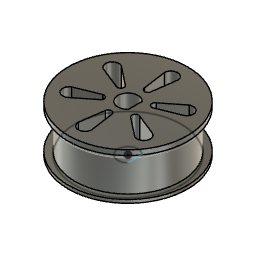
Maus_Komplettaufbau v3 (Autodesk Fusion 360 archive; units mm, degrees)
design "Wheel_v1"
Autodesk Fusion 360 part; units mm, degrees
sketch "Skizze1" plane through (0, 0, 0) normal (0, 0, 1) x (1, 0, 0)
  line L0 (1.05, 0) -> (1.05, 1.0712)
  line L1 (1.05, 0) -> (1.05, -1.0712)
  arc A0 (1.05, 1.0712) -> (1.05, -1.0712) centre (0, 0) ccw
  circle A1 centre (0, 0) radius 8
  dimension "d1" = 3
  dimension "d2" = 1.05
  dimension "d5" = 16
  constraint coincident A0.centre A1.centre
  measures "d1" diameter of A0
  measures "d2" distance of A0.centre L0.start
  measures "d5" diameter of A1
sketch "Skizze2" plane through (0, 0, 0) normal (0, 0, 1) x (1, 0, 0)
extrude "Extrusion2" add sketch "Skizze1" along normal blind 6
sketch "Skizze3" plane through (0, 0, 6) normal (0, 0, 1) x (-1, 0, 0)
  line L0 (-1.05, -1.0712) -> (-1.05, 1.0712)
  arc A0 (-1.05, -1.0712) -> (-1.05, 1.0712) centre (0, 0) ccw
  circle A1 centre (0, 0) radius 8
  line L1 (0.5, -3) -> (1, -6.5)
  line L2 (-1, -6.4999) -> (-0.4951, -2.93)
  arc A2 (-0.9608, -6.2227) -> (0.96, -6.22) centre (0, -6.5) ccw
  arc A3 (0.5, -3) -> (-0.4951, -2.93) centre (0, -3) ccw
  constraint coincident L1.end A2
  constraint coincident L2.start A2
  constraint tangent L2 A3
  constraint coincident L1 A2.end
  constraint coincident L2 A2.start
extrude "Extrusion3" cut sketch "Skizze3" against normal blind 6 contours L1 L2 A2 A3
pattern_circular "C-Anordnung1" count 6 over 360 about axis through (0, 0, 1.75) along (0, 0, 1) of "Extrusion3"
sketch "Skizze4" plane through (0, 0, 0) normal (0, 1, 0) x (1, 0, 0)
  line L0 (8, 0) -> (9, 0)
  line L1 (9, 0) -> (9, -0.5)
  line L2 (9, -0.5) -> (8, -0.5)
  line L3 (8, -0.5) -> (8, 0)
  line L4 (8, -6) -> (9, -6)
  line L5 (9, -6) -> (9, -5.5)
  line L6 (9, -5.5) -> (8, -5.5)
  line L7 (8, -5.5) -> (8, -6)
  constraint horizontal L0
  constraint vertical L1
  constraint horizontal L2
  constraint vertical L3
  constraint horizontal L4
  constraint vertical L5
  constraint horizontal L6
  constraint vertical L7
revolve "Drehen1" add sketch "Skizze4" angle 360 about axis through (0, 0, 1.75) along (0, 0, 1)
sketch "Skizze5" plane through (0, 0, 6) normal (0, 0, 1) x (-1, 0, 0)
  circle A0 centre (0, 0) radius 9
  arc A1 (-2.3481, -1.933) -> (-2.785, -1.0362) centre (-2.5981, -1.5) ccw
  line L0 (-2.3481, -1.933) -> (-5.1292, -4.116)
  arc A2 (-6.1291, -2.3839) -> (-5.1292, -4.116) centre (-5.6292, -3.25) ccw
  line L1 (-6.1291, -2.3839) -> (-2.785, -1.0362)
  arc A3 (-2.8481, 1.067) -> (-2.2899, 1.8937) centre (-2.5981, 1.5) ccw
  line L2 (-2.8481, 1.067) -> (-6.1292, 2.384)
  arc A4 (-5.1291, 4.116) -> (-6.1292, 2.384) centre (-5.6292, 3.25) ccw
  line L3 (-5.1291, 4.116) -> (-2.2899, 1.8937)
  arc A5 (-0.5, 3) -> (0.4951, 2.93) centre (0, 3) ccw
  line L4 (-0.5, 3) -> (-1, 6.5)
  arc A6 (1, 6.4999) -> (-1, 6.5) centre (0, 6.5) ccw
  line L5 (1, 6.4999) -> (0.4951, 2.93)
  arc A7 (2.3481, 1.933) -> (2.785, 1.0362) centre (2.5981, 1.5) ccw
  line L6 (2.3481, 1.933) -> (5.1292, 4.116)
  arc A8 (6.1291, 2.3839) -> (5.1292, 4.116) centre (5.6292, 3.25) ccw
  line L7 (6.1291, 2.3839) -> (2.785, 1.0362)
  arc A9 (2.8481, -1.067) -> (2.2899, -1.8937) centre (2.5981, -1.5) ccw
  line L8 (2.8481, -1.067) -> (6.1292, -2.384)
  arc A10 (5.1291, -4.116) -> (6.1292, -2.384) centre (5.6292, -3.25) ccw
  line L9 (5.1291, -4.116) -> (2.2899, -1.8937)
  arc A11 (0.5, -3) -> (-0.4951, -2.93) centre (0, -3) ccw
  line L10 (0.5, -3) -> (1, -6.5)
  arc A12 (-1, -6.4999) -> (1, -6.5) centre (0, -6.5) ccw
  line L11 (-1, -6.4999) -> (-0.4951, -2.93)
  line L12 (-1.05, -1.0712) -> (-1.05, 1.0712)
  arc A13 (-1.05, -1.0712) -> (-1.05, 1.0712) centre (0, 0) ccw
  line L13 (-1.1, 0) -> (-1.1, -1.0562)
  line L14 (-1.1, 0) -> (-1.1, 1.0562)
  arc A14 (-1.1, -1.0562) -> (-1.1, 1.0562) centre (0, 0) ccw
  dimension "d13" = 3.05
  constraint concentric A0 A14
  measures "d13" diameter of A14
extrude "Extrusion4" cut sketch "Skizze5" against normal blind 6 contours L13 L14 A14
extrude "Extrusion5" add 2 faces at (8.6332, -0.4471, 6) (5.0354, -0.3557, 6) along direction (0, 0, 1) blind 1
fillet "Abrundung1" radius 0.75 1 edges at (-8.3909, -3.2545, 5.5)

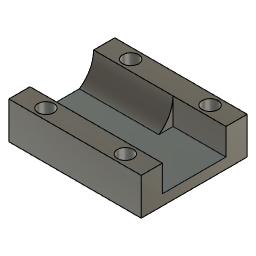
design "Motorhalter_v1"
Autodesk Fusion 360 part; units mm, degrees
sketch "Skizze1" plane through (0, 0, 0) normal (0, 0, 1) x (1, 0, 0)
  line L0 (0, 0) -> (-25, 0)
  line L1 (-25, 0) -> (-25, 20)
  line L2 (-25, 20) -> (0, 20)
  line L3 (0, 20) -> (0, 0)
  constraint horizontal L0
  constraint vertical L1
  constraint horizontal L2
  constraint vertical L3
  constraint coincident L0.start L3.end
extrude "Extrusion1" add sketch "Skizze1" along normal blind 7
sketch "Skizze2" plane through (0, 0, 0) normal (1, 0, 0) x (0, 1, 0)
  line L0 (0, 0) -> (20, 0)
  line L1 (20, 0) -> (20, 7)
  line L2 (20, 7) -> (0, 7)
  line L3 (0, 7) -> (0, 0)
  line L4 (10, 7) -> (4, 7)
  line L5 (4, 7) -> (4, 2)
  line L6 (4, 2) -> (16, 2)
  line L7 (16, 2) -> (16, 7)
  line L8 (16, 7) -> (10, 7)
  constraint midpoint L2 L4.start
  constraint coincident L2 L4.end
  constraint perpendicular L4 L5
  constraint coincident L2 L7.end
  constraint perpendicular L2 L7
extrude "Extrusion2" cut sketch "Skizze2" against normal blind 10 contours L2 L4 L5 L6 L7 L8
sketch "Skizze3" plane through (-10, 0, 0) normal (1, 0, 0) x (0, 1, 0)
  line L0 (16, 7) -> (4, 7)
  line L1 (4, 7) -> (4, 2)
  line L2 (4, 2) -> (16, 2)
  line L3 (16, 2) -> (16, 7)
  line L4 (6.6834, 2) -> (13.3166, 2)
  line L5 (16, 7) -> (4, 7)
  arc A0 (4, 7) -> (6.6834, 2) centre (10, 7) ccw
  arc A1 (13.3166, 2) -> (16, 7) centre (10, 7) ccw
  constraint midpoint L0 A0.centre
  constraint coincident L2 L4.start
  constraint coincident L4.end A0
  constraint coincident L2 L4.end
  constraint coincident L0.start L3.end
  constraint coincident L0.end L1.start
  constraint concentric A0 A1
extrude "Extrusion3" cut sketch "Skizze3" against normal blind 15 contours L0 L2 L4 L5 A0 A1
sketch "Skizze4" plane through (0, 0, 7) normal (0, 0, 1) x (-1, 0, 0)
  line L0 (10, -4) -> (25, -4)
  line L1 (25, -4) -> (25, 0)
  line L2 (25, 0) -> (0, 0)
  line L3 (0, 0) -> (0, -4)
  line L4 (0, -4) -> (10, -4)
  circle A0 centre (20, -2) radius 1.5
  circle A1 centre (5, -2) radius 1.5
  dimension "d7" = 3
  dimension "d8" = 3
  measures "d7" diameter of A0
  measures "d8" diameter of A1
extrude "Extrusion4" cut sketch "Skizze4" against normal blind 7 contours A0 | A1
sketch "Skizze5" plane through (0, 0, 2) normal (0, 0, 1) x (-1, 0, 0)
  line L0 (0, -4) -> (0, -16)
  line L1 (0, -16) -> (10, -16)
  line L2 (10, -16) -> (10, -13.3166)
  line L3 (10, -13.3166) -> (25, -13.3166)
  line L4 (25, -13.3166) -> (25, -6.6834)
  line L5 (25, -6.6834) -> (10, -6.6834)
  line L6 (10, -6.6834) -> (10, -4)
  line L7 (10, -4) -> (0, -4)
sketch "Skizze6" plane through (0, 0, 7) normal (0, 0, 1) x (-1, 0, 0)
  line L0 (25, -16) -> (10, -16)
  line L1 (10, -16) -> (0, -16)
  line L2 (0, -16) -> (0, -20)
  line L3 (0, -20) -> (25, -20)
  line L4 (25, -20) -> (25, -16)
  circle A0 centre (5, -18) radius 1.5
  circle A1 centre (20, -18) radius 1.5
  dimension "d11" = 3
  dimension "d12" = 3
  measures "d11" diameter of A0
  measures "d12" diameter of A1
extrude "Extrusion5" cut sketch "Skizze6" against normal blind 7 contours A0 | A1
